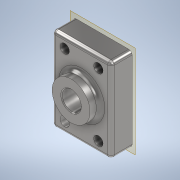
# Autodesk Inventor part: Фланецгайка_CPY
Saved by Autodesk Inventor 2021 (Build 250183000, 183)
## iProperties
Created: 2020-12-01
Part Number: Фланецгайка_CPY
Material: Сталь, углеродистая
Document SubType Name: Modeling
Designer: Тимоха
Mass: 8696.9 g
Surface Area: 893.705 cm^2
Volume: 1107.89 cm^3
Density: 7.85 g/cm^3
Appearance: С умеренной полировкой
Author: Тимоха
Autodesk Inventor part; units mm, degrees
ref_plane "YZ Plane" through (0, 0, 0) normal (1, 0, 0) x (0, 1, 0)
ref_plane "XZ Plane" through (0, 0, 0) normal (0, 1, 0) x (-1, 0, 0)
ref_plane "XY Plane" through (0, 0, 0) normal (0, 0, 1) x (1, 0, 0)
ref_plane "РабПлоскость1" through (0, 0, 0) normal (0, 0, 1) x (1, 0, 0)
sketch "Эскиз1" plane through (0, 0, 0) normal (0, 0, 1) x (1, 0, 0)
  line L0 (-70, -92) -> (-70, 92)
  line L1 (-62, 100) -> (62, 100)
  line L2 (70, 92) -> (70, -92)
  line L3 (62, -100) -> (-62, -100)
  line L4 (-70, -100) -> (70, 100) construction
  line L5 (-70, 100) -> (70, -100) construction
  arc A0 (-62, 100) -> (-70, 92) centre (-62, 92) ccw
  arc A1 (-70, -92) -> (-62, -100) centre (-62, -92) ccw
  arc A2 (62, -100) -> (70, -92) centre (62, -92) ccw
  arc A3 (70, 92) -> (62, 100) centre (62, 92) ccw
  line L6 (0, 75) -> (-40, 75)
  line L7 (-40, 75) -> (40, 75)
  line L8 (40, 75) -> (40, -75)
  line L9 (40, -75) -> (-40, -75)
  line L10 (-40, -75) -> (-40, 75)
  circle A4 centre (-40, 75) radius 11
  circle A5 centre (40, 75) radius 11
  circle A6 centre (-40, -75) radius 11
  circle A7 centre (40, -75) radius 11
  point P0 (0, 0)
  point P1 (0, 0)
  dimension "d24" = 200
  dimension "d25" = 140
  dimension "d26" = 8
  dimension "d27" = 8
  dimension "d28" = 8
  dimension "d29" = 8
  dimension "d31" = 40
  dimension "d32" = 80
  dimension "d33" = 150
  dimension "d34" = 22
  dimension "d35" = 22
  dimension "d36" = 22
  dimension "d37" = 22
  constraints: 22 end point, 8 centre point, 8 point on circle, 8 point on line, 8 tangent, 4 coincident, 4 parallel, 2 horizontal, 2 midpoint, 2 perpendicular
  measures "d24" distance of L4.start L5.start
  measures "d25" distance of L5.start L4.end
  measures "d26" radius of A0
  measures "d27" radius of A1
  measures "d28" radius of A2
  measures "d29" radius of A3
  measures "d31" distance of L6.start L6.end
  measures "d32" distance of L8.end L9.end
  measures "d33" distance of L7.end L8.end
  measures "d34" diameter of A4
  measures "d35" diameter of A5
  measures "d36" diameter of A6
  measures "d37" diameter of A7
extrude "Выдавливание1" add sketch "Эскиз1" along normal blind 50 contours L0 A0 L1 A3 L2 A2 L3 A1 | L7 A5 L8 A7 L9 A6 L10 A4 L6
sketch "Эскиз2" plane through (0, 0, 0) normal (0, 0, -1) x (-1, 0, 0)
  circle A0 centre (0, 0) radius 50
  dimension "d2" = 100
  constraints: 1 centre point, 1 coincident
  measures "d2" diameter of A0
extrude "Выдавливание2" add sketch "Эскиз2" along normal blind 15
sketch "Эскиз3" plane through (0, 0, 50) normal (0, 0, 1) x (1, 0, 0)
  circle A0 centre (0, 0) radius 45
  dimension "d5" = 90
  constraints: 1 centre point, 1 coincident
  measures "d5" diameter of A0
extrude "Выдавливание3" add sketch "Эскиз3" along normal blind 25
fillet "Сопряжение1" radius 10 1 edges at (-45, 0, 50)
sketch "Эскиз4" plane through (0, 0, 75) normal (0, 0, 1) x (1, 0, 0)
  circle A0 centre (0, 0) radius 55 projected
  circle A1 centre (0, 0) radius 22.5
  dimension "d9" = 45
  constraints: 1 centre point, 1 coincident
  measures "d9" diameter of A1
extrude "Выдавливание4" cut sketch "Эскиз4" against normal through all contours A1
chamfer "Фаска1" distance 2 angle 45 3 edges at (-22.5, 0, 75) (50, 0, -15) (-22.5, 0, -15)
sketch "Эскиз5" plane through (0, 0, 0) normal (1, 0, 0) x (0, 1, 0)
  line L0 (-24.5, -15) -> (24.5, -15) projected
  line L1 (48, -15) -> (-48, -15) projected
  line L2 (22.5, 73) -> (22.5, -13) projected
  line L3 (22.5, -15) -> (22.5, -8)
  line L4 (22.5, -8) -> (27.5, -8)
  line L5 (27.5, -8) -> (29.3756, -15)
  line L6 (0, -32.6) -> (0, 90.6) projected
  point P0 (0, 0)
  dimension "d15" = 7
  dimension "d16" = 5
  dimension "d17" = 105
  constraints: 6 end point, 3 point on line, 1 perpendicular
  measures "d15" distance of L3.start L3.end
  measures "d16" distance of L3.end L4.end
  measures "d17" angle of L4 L5
revolve "Вращение1" cut sketch "Эскиз5" angle 360 about axis through (0, 0, -10) along (0, 0, 1)
chamfer "Фаска2" distance 2 angle 45 1 edges at (-22.5, 0, -8)
fillet "Сопряжение2" radius 8 8 edges at (67.6569, 97.6569, 50) (0, 100, 50) (-67.6569, 97.6569, 50) (-70, 0, 50) (-67.6569, -97.6569, 50) (0, -100, 50) (67.6569, -97.6569, 50) (70, 0, 50)
